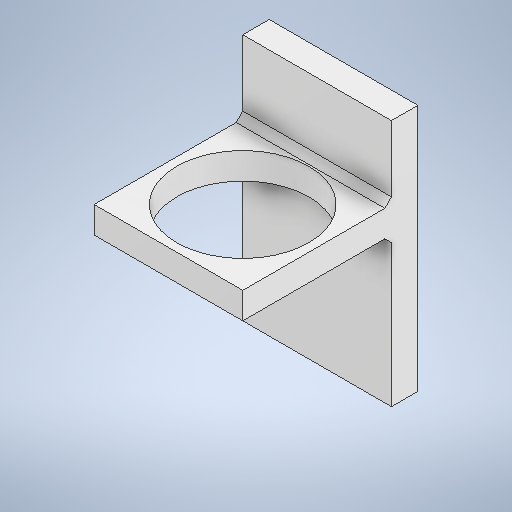
# Autodesk Inventor part: Air Filter Bracket
Saved by Autodesk Inventor 2025 (Build 290162000, 162)
## iProperties
Created: 2025-08-21
Part Number: Air Filter Bracket
Material: Acetal Resin, White
Document SubType Name: Modeling
Designer: Caleb Fangmeier
Density: 1.425 g/cm^3
Appearance: Smooth - White
Author: Caleb Fangmeier
Autodesk Inventor part; units mm, degrees
ref_plane "YZ Plane" through (0, 0, 0) normal (1, 0, 0) x (0, 1, 0)
ref_plane "XZ Plane" through (0, 0, 0) normal (0, 1, 0) x (-1, 0, 0)
ref_plane "XY Plane" through (0, 0, 0) normal (0, 0, 1) x (1, 0, 0)
sketch "Sketch1" plane through (0, 0, 0) normal (0, 1, 0) x (-1, 0, 0)
  line L0 (-22.5, 22.5) -> (22.5, 22.5)
  line L1 (22.5, 22.5) -> (22.5, -22.5)
  line L2 (22.5, -22.5) -> (-22.5, -22.5)
  line L3 (-22.5, -22.5) -> (-22.5, 22.5)
  line L4 (-22.5, 22.5) -> (22.5, -22.5) construction
  line L5 (22.5, 22.5) -> (-22.5, -22.5) construction
  circle A0 centre (0, 0) radius 20
  dimension "d0" = 40
  dimension "d1" = 45
  dimension "d2" = 45
  constraints: 12 end point, 2 midpoint, 2 parallel, 1 centre point, 1 coincident, 1 horizontal, 1 perpendicular
  measures "d0" diameter of A0
  measures "d1" distance of L1.end L2.end
  measures "d2" distance of L0.end L1.end
extrude "Extrusion1" add sketch "Sketch1" along normal blind 8
sketch "Sketch2" plane through (22.5, 0, -22.5) normal (0, 0, -1) x (-1, 0, 0)
  line L0 (0, 0) -> (45, 0) projected
  line L1 (45, 0) -> (0, 0)
  line L2 (0, 0) -> (0, 30)
  line L3 (0, 30) -> (45, 30)
  line L4 (45, 30) -> (45, 0)
  line L5 (45, 0) -> (0, 0)
  line L6 (0, 0) -> (0, -45)
  line L7 (0, -45) -> (45, -45)
  line L8 (45, -45) -> (45, 0)
  point P0 (22.5, 0)
  dimension "d5" = 30
  dimension "d8" = 45
  constraints: 16 end point, 4 parallel, 2 horizontal, 2 perpendicular, 1 point on line
  measures "d5" distance of L1.end L2.end
  measures "d8" distance of L0.start L6.end
extrude "Extrusion2" add sketch "Sketch2" along normal blind 8
chamfer "Chamfer1" distance 2 angle 45 2 edges at (0, 8, -22.5) (0, 0, -22.5)
body "Solid1"
